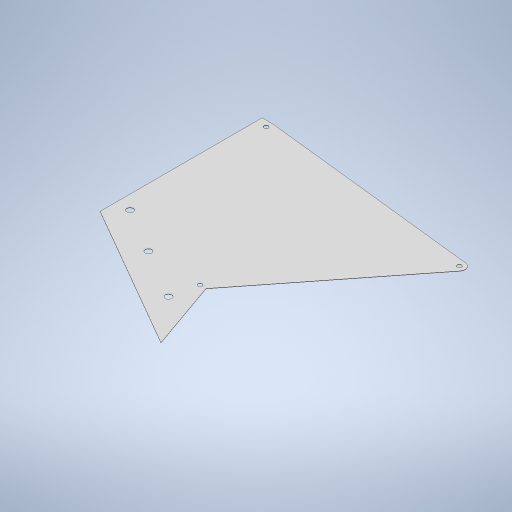
# Autodesk Inventor part: base_main_pcb_p1_itr3
Saved by Autodesk Inventor 2024 (Build 280153000, 153)
## iProperties
Created: 2026-03-21
Part Number: base_main_pcb_p1_itr3
Material: Generic
Document SubType Name: Modeling
Designer: schar
Density: 1 g/cm^3
Appearance: Default
Author: schar
Autodesk Inventor part; units mm, degrees
ref_plane "YZ Plane" through (0, 0, 0) normal (1, 0, 0) x (0, 1, 0)
ref_plane "XZ Plane" through (0, 0, 0) normal (0, 1, 0) x (-1, 0, 0)
ref_plane "Work Plane1" through (-205, 2.2, 290) normal (0, 1, 0) x (1, 0, 0)
sketch "Sketch1" plane through (-205, 2.2, 290) normal (0, 1, 0) x (1, 0, 0)
  line L0 (0, 277.1478) -> (0, 0)
  line L1 (0, 172.4077) -> (101.9371, 112.2551)
  line L2 (138.3655, 8.2698) -> (91, 143.475)
  line L3 (0, 154.0621) -> (109.4535, 90.7992)
  circle A0 centre (10.5733, 166.1684) radius 2.5
  circle A1 centre (44.6303, 146.0715) radius 2.5
  circle A2 centre (82.1326, 123.9416) radius 2.5
  circle A3 centre (86.5, 143.475) radius 1.675
  circle A4 centre (86.5, 143.475) radius 1.675
  circle A5 centre (86.5, 143.475) radius 1.675
  circle A6 centre (86.5, 143.475) radius 1.675
  line L4 (91, 143.475) -> (176.0383, 251.6946)
  line L5 (91, 143.475) -> (176.0383, 251.6946)
  line L6 (91, 143.475) -> (176.0383, 251.6946)
  line L7 (91, 143.475) -> (176.0383, 251.6946)
  circle A7 centre (172.5, 254.475) radius 1.675
  circle A8 centre (172.5, 254.475) radius 1.675
  circle A9 centre (172.5, 254.475) radius 1.675
  circle A10 centre (172.5, 254.475) radius 1.675
  arc A11 (176.0383, 251.6946) -> (172.5, 258.975) centre (172.5, 254.475) ccw
  arc A12 (176.0383, 251.6946) -> (172.5, 258.975) centre (172.5, 254.475) ccw
  arc A13 (176.0383, 251.6946) -> (172.5, 258.975) centre (172.5, 254.475) ccw
  arc A14 (176.0383, 251.6946) -> (172.5, 258.975) centre (172.5, 254.475) ccw
  line L8 (172.5, 258.975) -> (7.9941, 277.1478)
  line L9 (172.5, 258.975) -> (7.9941, 277.1478)
  line L10 (172.5, 258.975) -> (7.9941, 277.1478)
  line L11 (172.5, 258.975) -> (7.9941, 277.1478)
  circle A15 centre (7.5, 272.675) radius 1.675
  circle A16 centre (7.5, 272.675) radius 1.675
  circle A17 centre (7.5, 272.675) radius 1.675
  circle A18 centre (7.5, 272.675) radius 1.675
  line L12 (7.9941, 277.1478) -> (0, 277.1478)
  line L13 (7.9941, 277.1478) -> (0, 277.1478)
  line L14 (7.9941, 277.1478) -> (0, 277.1478)
  line L15 (7.9941, 277.1478) -> (0, 277.1478)
  point P0 (205, 290)
extrude "Extrusion1" add sketch "Sketch1" along normal blind 0.2 contours L12 L8 A11 L4 L2 L1 A2 A1 A0 L0 | L1 A0 A1 A2 L2 L3 L0
body "Solid2"
